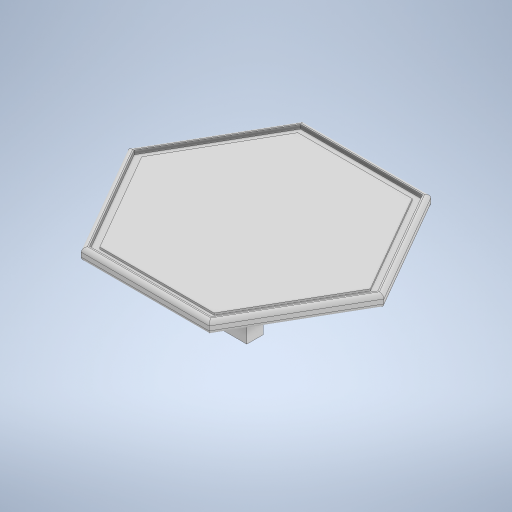
# Autodesk Inventor part: OV-PAM_n_6_bottom
Saved by Autodesk Inventor 2024 (Build 280153000, 153)
## iProperties
Created: 2023-08-31
Part Number: OV-PAM_n_6_bottom
Material: 일반
Document SubType Name: Modeling
Designer: jsw
Density: 1 g/cm^3
Appearance: 기본값
Author: jsw
Autodesk Inventor part; units mm, degrees
ref_plane "YZ Plane" through (0, 0, 0) normal (1, 0, 0) x (0, 1, 0)
ref_plane "XZ Plane" through (0, 0, 0) normal (0, 1, 0) x (-1, 0, 0)
ref_plane "XY Plane" through (0, 0, 0) normal (0, 0, 1) x (1, 0, 0)
sketch "스케치1" plane through (0, 0, 0) normal (0, 1, 0) x (-1, 0, 0)
  line L0 (17.6385, -30.5508) -> (-17.6385, -30.5508)
  line L1 (-17.6385, -30.5508) -> (-35.277, 0)
  line L2 (-35.277, 0) -> (-17.6385, 30.5508)
  line L3 (-17.6385, 30.5508) -> (17.6385, 30.5508)
  line L4 (17.6385, 30.5508) -> (35.277, 0)
  line L5 (35.277, 0) -> (17.6385, -30.5508)
  line L6 (19.486, -33.7508) -> (-19.486, -33.7508)
  line L7 (-19.486, -33.7508) -> (-38.972, 0)
  line L8 (-38.972, 0) -> (-19.486, 33.7508)
  line L9 (-19.486, 33.7508) -> (19.486, 33.7508)
  line L10 (19.486, 33.7508) -> (38.972, 0)
  line L11 (38.972, 0) -> (19.486, -33.7508)
  point P0 (0, 0)
  point P1 (0, 0)
  point P2 (0, 0)
  dimension "d0" = 70.554
  dimension "d1" = 3.2
  constraints: 24 end point, 2 coincident, 2 horizontal, 26 other
  measures "d0" distance of L2.end L0.start
  measures "d1" distance between parallel lines of L0 L6
extrude "돌출1" add sketch "스케치1" along normal blind 3.7 contours L0 L1 L2 L3 L4 L5 | L6 L7 L8 L9 L10 L11
sketch "스케치2" plane through (0, 3.7, 0) normal (0, 1, 0) x (1, 0, 0)
  line L0 (-18.5623, 32.1508) -> (18.5623, 32.1508)
  line L1 (18.5623, 32.1508) -> (37.1245, 0)
  line L2 (37.1245, 0) -> (18.5623, -32.1508)
  line L3 (18.5623, -32.1508) -> (-18.5623, -32.1508)
  line L4 (-18.5623, -32.1508) -> (-37.1245, 0)
  line L5 (-37.1245, 0) -> (-18.5623, 32.1508)
  line L6 (-19.486, 33.7508) -> (-38.972, 0) projected
  point P0 (0, 0)
  point P1 (0, 0)
  dimension "d4" = 1.6
  constraints: 12 end point, 1 coincident, 1 horizontal, 13 other
  measures "d4" distance between parallel lines of L5 L6
extrude "돌출2" cut sketch "스케치2" against normal blind 1.2
sketch "스케치3" plane through (0, 2.5, 0) normal (0, 1, 0) x (1, 0, 0)
  line L0 (17.4076, -30.1508) -> (-17.4076, -30.1508)
  line L1 (-17.4076, -30.1508) -> (-34.8151, 0)
  line L2 (-34.8151, 0) -> (-17.4076, 30.1508)
  line L3 (-17.4076, 30.1508) -> (17.4076, 30.1508)
  line L4 (17.4076, 30.1508) -> (34.8151, 0)
  line L5 (34.8151, 0) -> (17.4076, -30.1508)
  line L6 (-18.5623, 32.1508) -> (18.5623, 32.1508) projected
  point P0 (0, 0)
  point P1 (0, 0)
  dimension "d7" = 2
  constraints: 12 end point, 1 coincident, 1 horizontal, 13 other
  measures "d7" distance between parallel lines of L6 L3
extrude "돌출3" add sketch "스케치3" along normal blind 0.6
fillet "모깎기1" radius 1.2 12 edges at (0, 3.7, -33.7508) (0, 0, -33.7508) (-29.229, 3.7, -16.8754) (-29.229, 0, -16.8754) (-29.229, 3.7, 16.8754) (-29.229, 0, 16.8754) (0, 0, 33.7508) (0, 3.7, 33.7508) (29.229, 0, 16.8754) (29.229, 3.7, 16.8754) (29.229, 3.7, -16.8754) (29.229, 0, -16.8754)
sketch "스케치10" plane through (0, 0, 0) normal (0, -1, 0) x (1, 0, 0)
  line L0 (-12.5, 15.3) -> (12.5, 15.3)
  line L1 (12.5, 15.3) -> (12.5, 10.3)
  line L2 (12.5, 10.3) -> (-12.5, 10.3)
  line L3 (-12.5, 10.3) -> (-12.5, 15.3)
  line L4 (-12.5, 15.3) -> (12.5, 10.3) construction
  line L5 (12.5, 15.3) -> (-12.5, 10.3) construction
  line L6 (0, 0) -> (7.4968, 0)
  line L7 (-12.5, -15.3) -> (12.5, -15.3)
  line L8 (12.5, -15.3) -> (12.5, -10.3)
  line L9 (12.5, -10.3) -> (-12.5, -10.3)
  line L10 (-12.5, -10.3) -> (-12.5, -15.3)
  line L11 (-12.5, -15.3) -> (12.5, -10.3) construction
  line L12 (12.5, -15.3) -> (-12.5, -10.3) construction
  point P0 (0, 12.8)
  point P1 (0, -12.8)
  dimension "d51" = 25
  dimension "d52" = 5
  dimension "d53" = 10.3
  constraints: 26 end point, 5 symmetric about line, 2 horizontal, 2 midpoint, 2 parallel, 1 perpendicular, 1 vertical alignment
  measures "d51" distance of L0.start L0.end
  measures "d52" distance of L0.end L1.end
  measures "d53" distance from line of L6.start L2
extrude "돌출7" add sketch "스케치10" along normal blind 15
sketch "스케치11" plane through (12.5, 0, -15.3) normal (0, 0, -1) x (-1, 0, 0)
  circle A0 centre (7.5, -7.5) radius 1.25
  line L0 (-6.2932, 0) -> (31.2932, 0) projected
  line L1 (12.5, 0) -> (12.5, -3.2028)
  circle A1 centre (17.5, -7.5) radius 1.25
  point P0 (12.5, 0)
  dimension "d56" = 2.5
  dimension "d57" = 7.5
  dimension "d58" = 5
  constraints: 2 centre point, 2 end point, 1 midpoint, 1 symmetric about line, 1 vertical, 1 other
  measures "d56" diameter of A0
  measures "d57" distance from line of A0.centre L0
  measures "d58" horizontal distance of L1.start A0.centre
extrude "돌출8" cut sketch "스케치11" against normal up to surface (30.6 mm away)
